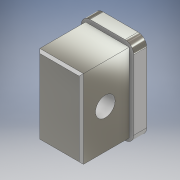
# Autodesk Inventor part: reverse gear steam chest side valve
Saved by Autodesk Inventor 2017 (Build 210142000, 142)
## iProperties
Created: 2018-11-06
Part Number: reverse gear steam chest side valve
Material: Generic
Document SubType Name: Modeling
Designer: User
Density: 1 g/cm^3
Appearance: Default
Author: User
Autodesk Inventor part; units mm, degrees
ref_plane "YZ Plane" through (0, 0, 0) normal (1, 0, 0) x (0, 1, 0)
ref_plane "XZ Plane" through (0, 0, 0) normal (0, 1, 0) x (-1, 0, 0)
ref_plane "XY Plane" through (0, 0, 0) normal (0, 0, 1) x (1, 0, 0)
sketch "Sketch1" plane through (0, 0, 0) normal (0, 1, 0) x (-1, 0, 0)
  line L0 (0, 0) -> (-12, 0)
  line L1 (-12, 0) -> (-12, -20)
  line L2 (-12, -20) -> (0, -20)
  line L3 (0, -20) -> (0, 0)
  line L4 (-6, 0) -> (-6, -1)
  line L5 (-6, -1) -> (-1, -1)
  line L6 (-1, -1) -> (-11, -1)
  line L7 (-11, -1) -> (-11, -19)
  line L8 (-11, -19) -> (-1, -19)
  line L9 (-1, -19) -> (-1, -1)
  dimension "d0" = 12
  dimension "d1" = 20
  dimension "d2" = 1
  dimension "d3" = 5
  dimension "d4" = 10
  dimension "d5" = 18
  dimension "d35" = 0
  dimension "d36" = 1
  constraints: 20 end point, 4 perpendicular, 2 horizontal, 2 parallel, 1 midpoint, 1 point on line, 1 vertical
  measures "d0" distance of L2.end L1.end
  measures "d1" distance of L1.end L0.end
  measures "d2" distance of L4.start L4.end
  measures "d3" distance of L4.end L5.end
  measures "d4" distance of L5.end L6.end
  measures "d5" distance of L6.end L7.end
  measures "d35" distance from line of point (0, 0) L3
  measures "d36" distance from line of point (0, 0) L5
extrude "Extrusion1" add sketch "Sketch1" along normal blind 3
sketch "Sketch2" plane through (0, 3, 0) normal (0, 1, 0) x (1, 0, 0)
  line L0 (11, 1) -> (1, 1)
  line L1 (11, 19) -> (11, 1)
  line L2 (1, 1) -> (11, 1)
  line L3 (11, 1) -> (11, 19)
  line L4 (11, 19) -> (1, 19)
  line L5 (1, 19) -> (1, 1)
  point P0 (0, 0)
  point P1 (0, 0)
  dimension "d37" = 10
  dimension "d38" = 18
  dimension "d39" = 11
  dimension "d40" = 19
  dimension "d41" = 11
  dimension "d42" = 1
  constraints: 12 end point, 4 parallel, 1 horizontal, 1 perpendicular
  measures "d37" distance between parallel lines of L3 L5
  measures "d38" distance between parallel lines of L4 L0
  measures "d39" distance from line of point (0, 0) L3
  measures "d40" distance from line of point (0, 0) L4
  measures "d41" distance from line of point (0, 0) L3
  measures "d42" distance from line of point (0, 0) L0
extrude "Extrusion4" add sketch "Sketch2" against normal blind 14
sketch "Sketch5" plane through (11, -11, -1) normal (1, 0, 0) x (0, 0, -1)
  line L0 (0, 11) -> (18, 11) projected
  line L1 (0, 11) -> (0, 0) projected
  line L2 (18, 0) -> (0, 0) projected
  line L3 (18, 11) -> (18, 0) projected
  circle A0 centre (9, 5.5) radius 2.25
  point P0 (-1, 11)
  dimension "d21" = 4.5
  dimension "d43" = 9
  dimension "d44" = 5.5
  constraints: 1 centre point
  measures "d21" diameter of A0
  measures "d43" distance from line of A0.centre L3
  measures "d44" distance from line of A0.centre L2
extrude "Extrusion5" cut sketch "Sketch5" against normal through all contours A0
sketch "Sketch6" plane through (0, 3, 0) normal (0, 1, 0) x (1, 0, 0)
  line L0 (6, 0) -> (6, 3)
  line L1 (6, 3) -> (6, 17)
  line L2 (6, 3) -> (3, 3)
  line L3 (3, 3) -> (3, 17)
  line L4 (3, 17) -> (9, 17)
  line L5 (9, 17) -> (9, 3)
  line L6 (9, 3) -> (6, 3)
  point P0 (0, 0)
  point P1 (0, 0)
  dimension "d24" = 3
  dimension "d25" = 14
  dimension "d26" = 3
  dimension "d27" = 6
  dimension "d28" = 14
  dimension "d29" = 9
  dimension "d30" = 3
  dimension "d31" = 9
  dimension "d32" = 3
  constraints: 14 end point, 4 perpendicular, 2 point on line, 1 horizontal, 1 vertical
  measures "d24" distance of L0.start L0.end
  measures "d25" distance of L0.end L1.end
  measures "d26" distance of L0.end L2.end
  measures "d27" distance of L3.end L4.end
  measures "d28" distance between parallel lines of L4 L6
  measures "d29" distance from line of point (0, 0) L5
  measures "d30" distance from line of point (0, 0) L6
  measures "d31" distance from line of point (0, 0) L5
  measures "d32" distance from line of point (0, 0) L6
extrude "Extrusion6" cut sketch "Sketch6" against normal blind 3
chamfer "Chamfer1" distance 0.5 angle 45 4 edges at (11, -11, -10) (1, -11, -10) (6, -11, -1) (6, -11, -19)
fillet "Fillet1" radius 2 4 edges at (12, 1.5, -20) (12, 1.5, 0) (0, 1.5, -20) (0, 1.5, 0)
fillet "Fillet2" radius 2 4 edges at (3, 1.5, -3) (3, 1.5, -17) (9, 1.5, -3) (9, 1.5, -17)
body "Solid1"
